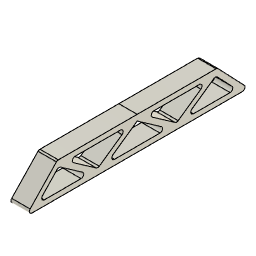
304 Beam v25 (Autodesk Fusion 360 design; units mm, degrees)
Autodesk Fusion 360 part; units mm, degrees
sketch "Sketch1" plane through (0, 0, 0) normal (1, 0, 0) x (0, 1, 0)
  line L0 (0, 0) -> (50, 0) construction
  line L1 (0, 0) -> (0, 21) construction
  line L2 (0, 21) -> (20, 21) construction
  line L3 (0, 0) -> (20, 21) construction
  line L4 (20, 21) -> (50, 0) construction
  line L5 (50, 0) -> (80, 0) construction
  line L6 (20, 21) -> (80, 21) construction
  line L7 (50, 0) -> (80, 21) construction
  line L8 (80, 0) -> (80, 21) construction
  line L9 (7.8851, 5.3793) -> (19.0759, 17.1297)
  line L10 (62.6895, 2) -> (80, 2)
  line L11 (9.3333, 2) -> (37.3105, 2)
  line L12 (31.5425, 15.3615) -> (48.8531, 3.2442)
  line L13 (21.6711, 17.3889) -> (38.4575, 5.6385)
  line L14 (61.5425, 5.6385) -> (80, 18.5587)
  line L15 (0, -2) -> (50, -2)
  line L16 (50, -2) -> (80, -2)
  line L17 (20, 23) -> (80, 23)
  line L18 (-1.4483, 1.3793) -> (18.5517, 22.3793)
  line L19 (32.6895, 19) -> (67.3105, 19)
  line L20 (51.1469, 3.2442) -> (68.4575, 15.3615)
  arc A0 (20, 23) -> (18.5517, 22.3793) centre (20, 21) ccw
  arc A1 (-1.4483, 1.3793) -> (0, -2) centre (0, 0) ccw
  arc A2 (21.6711, 17.3889) -> (19.0759, 17.1297) centre (20.5242, 15.7504) ccw
  arc A3 (7.8851, 5.3793) -> (9.3333, 2) centre (9.3333, 4) ccw
  arc A4 (37.3105, 2) -> (38.4575, 5.6385) centre (37.3105, 4) ccw
  arc A5 (32.6895, 19) -> (31.5425, 15.3615) centre (32.6895, 17) ccw
  arc A6 (68.4575, 15.3615) -> (67.3105, 19) centre (67.3105, 17) ccw
  arc A7 (48.8531, 3.2442) -> (51.1469, 3.2442) centre (50, 4.8826) ccw
  arc A8 (61.5425, 5.6385) -> (62.6895, 2) centre (62.6895, 4) ccw
  line L21 (80, 18.5587) -> (80, 23)
  line L22 (80, 2) -> (80, -2)
  dimension "d52" = 50
  dimension "d53" = 21
  dimension "d54" = 20
  dimension "d55" = 30
  dimension "d56" = 60
  dimension "d61" = 25
  dimension "d62" = 4
  dimension "d63" = 2
  dimension "d64" = 2
  dimension "d65" = 4
  dimension "d66" = 4
  dimension "d67" = 2
  dimension "d68" = 4
  dimension "d69" = 2
  dimension "d70" = 4
  dimension "d71" = 2
  dimension "d73" = 4
  dimension "d74" = 2
  dimension "d75" = 2
  dimension "d76" = 2
  dimension "d77" = 2
  dimension "d78" = 2
  dimension "d79" = 2
  dimension "d80" = 2
  dimension "d81" = 2
  dimension "d82" = 2
  constraint coincident L0.start L1.start
  constraint horizontal L0
  constraint perpendicular L0 L1
  constraint perpendicular L1 L2
  constraint parallel L0 L5
  constraint parallel L2 L6
  constraint parallel L4 L13
  constraint parallel L7 L14
  constraint parallel L4 L12
  constraint parallel L7 L20
  constraint parallel L3 L9
  constraint parallel L5 L10
  constraint parallel L0 L11
  constraint parallel L0 L15
  constraint parallel L5 L16
  constraint parallel L6 L17
  constraint parallel L3 L18
  constraint tangent L17 A0
  constraint tangent L18 A0
  constraint tangent L18 A1
  constraint tangent L15 A1
  constraint tangent L13 A2
  constraint tangent L9 A2
  constraint tangent L9 A3
  constraint tangent L11 A3
  constraint tangent L13 A4
  constraint tangent L11 A4
  constraint tangent L12 A5
  constraint tangent L19 A5
  constraint tangent L20 A6
  constraint tangent L19 A6
  constraint tangent L20 A7
  constraint tangent L12 A7
  constraint tangent L14 A8
  constraint tangent L10 A8
  constraint coincident L8 L14.end
  constraint perpendicular L17 L21
  constraint coincident L8 L10.end
  constraint perpendicular L16 L22
  measures "d52" distance of L0.start L0.end
  measures "d53" distance of L0.start L1.end
  measures "d54" distance of L1.end L2.end
  measures "d55" distance of L0.end L5.end
  measures "d56" distance of L2.end L6.end
  measures "d61" distance of L15 L17
  measures "d62" distance of L17 L19
  measures "d63" distance of L6 L17
  measures "d64" distance of L7 L14
  measures "d65" distance of L14 L20
  measures "d66" distance of L12 L13
  measures "d67" distance of L4 L12
  measures "d68" distance of L9 L18
  measures "d69" distance of L3 L9
  measures "d70" distance of L11 L15
  measures "d71" distance of L0 L11
  measures "d73" distance of L10 L16
  measures "d74" radius of A0
  measures "d75" radius of A1
  measures "d76" radius of A2
  measures "d77" radius of A3
  measures "d78" radius of A4
  measures "d79" radius of A5
  measures "d80" radius of A6
  measures "d81" radius of A7
  measures "d82" radius of A8
extrude "Extrude2" add sketch "Sketch1" along normal blind 14 makes body 1
ref_plane "WorkPlane1" through (0, 80, 0) normal (0, 1, 0) x (0, 0, 1)
mirror "Mirror1" about plane through (0, 80, 0) normal (0, 1, 0) of bodies 1 merged
copy_body "Body->Comp3" bodies 1 removing the originals makes body 2 in component "Truss Half"
component "Truss Half" placed x (1, 0, 0) y (0, 1, 0) z (0, 0, 1) at (0, 0, 0)
